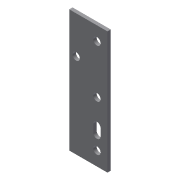
# Autodesk Inventor part: Clawplate
Saved by Autodesk Inventor 2015 (Build 190159000, 159)
## iProperties
Created: 2015-01-19
Part Number: Clawplate
Material: Generic
Document SubType Name: Sheet Metal
Designer: Tanner
Density: 1 g/cm^3
Sheet Metal Rule: Default
Appearance: Default
Author: Tanner
Autodesk Inventor part; units mm, degrees
ref_plane "YZ Plane" through (0, 0, 0) normal (1, 0, 0) x (0, 1, 0)
ref_plane "XZ Plane" through (0, 0, 0) normal (0, 1, 0) x (-1, 0, 0)
ref_plane "XY Plane" through (0, 0, 0) normal (0, 0, 1) x (1, 0, 0)
sketch "Sketch1" plane through (0, 0, 0) normal (0, 0, 1) x (1, 0, 0)
  line L0 (0, 0) -> (35.052, 0)
  line L1 (35.052, 0) -> (35.052, 112.1918)
  line L2 (35.052, 112.1918) -> (0, 112.1918)
  line L3 (0, 112.1918) -> (0, 0)
  dimension "d0" = 35.052
  dimension "d1" = 112.1918
  measures "d0" distance of L2.end L1.end
  measures "d1" distance of L1.end L0.end
extrude "Plate1" add sketch "Sketch1" along normal blind 3.048
sketch "Sketch2" plane through (0, 0, 3.048) normal (0, 0, 1) x (1, 0, 0)
  circle A0 centre (25.4, 99.4918) radius 3.3655
  circle A1 centre (25.4, 12.7603) radius 3.3655
  circle A2 centre (25.4, 55.0418) radius 3.3655
  circle A3 centre (6.35, 77.978) radius 3.3655
  line L0 (0, 0) -> (0, 112.1918) projected
  line L1 (28.7655, 32.1818) -> (28.7655, 25.4508)
  line L2 (22.0345, 25.4508) -> (22.0345, 32.1818)
  arc A4 (28.7655, 32.1818) -> (22.0345, 32.1818) centre (25.4, 32.1818) ccw
  line L3 (22.0345, 32.1818) -> (22.0345, 32.1818)
  line L4 (28.7655, 32.1818) -> (28.7655, 32.1818)
  arc A5 (22.0345, 25.4508) -> (28.7655, 25.4508) centre (25.4, 25.4508) ccw
  line L5 (0, 112.1918) -> (35.052, 112.1918) projected
  line L6 (35.052, 112.1918) -> (35.052, 0) projected
  point P0 (25.786, 22.1075)
  dimension "hole" = 6.731
  dimension "d42" = 6.731
  dimension "d43" = 6.731
  dimension "d44" = 6.731
  dimension "d49" = 25.4
  dimension "d50" = 6.35
  dimension "d51" = 25.4
  dimension "d54" = 25.4
  dimension "d55" = 44.45
  dimension "d58" = 22.0345
  dimension "d62" = 6.731
  dimension "d63" = 22.86
  dimension "d64" = 12.6905
  dimension "d66" = 25.4
  dimension "d67" = 25.4
  dimension "d68" = 12.7
  dimension "d69" = 21.5138
  dimension "d70" = 3.3655
  dimension "d75" = 9.3472
  dimension "d78" = 6.731
  dimension "d80" = 180
  dimension "d81" = 6.731
  constraints: 8 end point, 6 centre point, 5 point on circle, 2 horizontal, 2 perpendicular, 1 parallel, 1 tangent
  measures "hole" diameter of A0
  measures "d42" diameter of A3
  measures "d43" diameter of A2
  measures "d44" diameter of A1
  measures "d49" distance from line of L0 A0.centre
  measures "d50" distance from line of L0 A3.centre
  measures "d51" distance from line of L0 A2.centre
  measures "d54" distance from line of L0 A1.centre
  measures "d55" distance of A2.centre A0.centre
  measures "d58" distance between parallel lines of L0 L2
  measures "d62" distance of A4.centre A5.centre
  measures "d63" distance of A4.centre A2.centre
  measures "d64" distance of A1.centre A5.centre
  measures "d66" distance from line of L0 A4.centre
  measures "d67" distance from line of L0 A5.centre
  measures "d68" distance from line of L5 A0.centre
  measures "d69" vertical distance of A0.centre A3.centre
  measures "d70" radius of A4
  measures "d75" vertical distance of A1.centre point (25.786, 22.108)
  measures "d78" distance between parallel lines of L1 L2
  measures "d81" distance of L1.start L1.end
extrude "Extrusion1" cut sketch "Sketch2" against normal blind 25.4
equation "\"d42\" = hole"
equation "\"d43\" = hole"
equation "\"d44\" = hole"
equation "\"d70\" = 0.5 * hole"
equation "\"BendRadius\" = Thickness"
equation "\"BendReliefWidth\" = Thickness"
equation "\"BendReliefDepth\" = 0.5 * Thickness"
equation "\"CornerReliefSize\" = 4 * Thickness"
equation "\"MinimumRemnant\" = 2 * Thickness"
equation "\"TransitionRadius\" = BendRadius"
equation "\"JacobiRadiusSize\" = BendRadius"
equation "\"GapSize\" = Thickness"
equation "\"d2\" = BendRadius"
equation "\"Thickness\" = 3.048"
body "Solid1"
